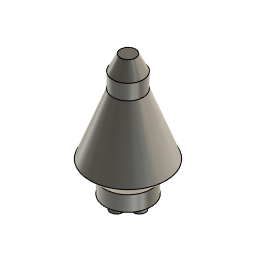
Orbiter v3 (Autodesk Fusion 360 design; units mm, degrees)
Autodesk Fusion 360 part; units mm, degrees
sketch "Sketch1" plane through (0, 0, 0) normal (0, 0, 1) x (1, 0, 0)
  circle A0 centre (0, 0) radius 1500
  constraint coincident A0.centre origin
extrude "Extrude2" add sketch "Sketch1" along normal mid plane 1000 makes body 1
sketch "Sketch4" plane through (0, 0, 0) normal (0, 1, 0) x (1, 0, 0)
  line L0 (0, -500) -> (-1500, -500)
  line L1 (-1500, -500) -> (-2500, -1500)
  line L2 (-2500, -1500) -> (0, -1500)
  line L3 (0, -1500) -> (0, -500)
  line L4 (0, 0) -> (0, -3000)
  constraint horizontal L0
  constraint parallel L0 L2
  constraint perpendicular L0 L3
  constraint coincident L4.start origin
  constraint perpendicular L0 L4
revolve "Revolve1" add sketch "Sketch4" angle 360 about axis through (0, 0, 0) along (0, 0, 1) bodies 1
sketch "Sketch5" plane through (0, 0, 0) normal (0, 1, 0) x (1, 0, 0)
  line L0 (0, -1500) -> (-2500, -1500)
  line L1 (-2500, -1500) -> (-1000, -5500)
  line L2 (-1000, -5500) -> (0, -5500)
  line L3 (0, -5500) -> (0, -1500)
  line L4 (0, 0) -> (0, -6500)
  constraint horizontal L0
  constraint parallel L0 L2
  constraint perpendicular L0 L3
  constraint coincident L4.start origin
  constraint perpendicular L2 L4
revolve "Revolve2" add sketch "Sketch5" angle 360 about axis through (0, 0, 0) along (0, 0, 1) bodies 1
sketch "Sketch6" plane through (0, 0, 5500) normal (0, 0, 1) x (-1, 0, 0)
  circle A0 centre (0, 0) radius 1000
  circle A1 centre (0, 0) radius 1000
  constraint coincident A0.centre A1.centre
extrude "Extrude3" add sketch "Sketch6" along normal blind 1000 bodies 1
sketch "Sketch7" plane through (0, 0, 0) normal (0, 1, 0) x (1, 0, 0)
  line L0 (0, -6500) -> (-1000, -6500)
  line L1 (-1000, -6500) -> (-500, -7500)
  line L2 (-500, -7500) -> (0, -7500)
  line L3 (0, -7500) -> (0, -6500)
  line L4 (0, -6500) -> (0, -8000)
  constraint horizontal L0
  constraint parallel L0 L2
  constraint perpendicular L0 L3
  constraint perpendicular L0 L4
revolve "Revolve3" add sketch "Sketch7" angle 360 about axis through (0, 0, 6500) along (0, 0, 1) bodies 1
sketch "Sketch8" plane through (0, 0, 0) normal (0, 1, 0) x (1, 0, 0)
sketch "Sketch9" plane through (0, 0, 0) normal (0, 1, 0) x (1, 0, 0)
  line L0 (-1000, 500) -> (-500, 500)
  line L1 (-500, 500) -> (-350, 1000)
  line L2 (-350, 1000) -> (-1150, 1000)
  line L3 (-1150, 1000) -> (-1000, 500)
  line L4 (-750, 0) -> (-750, 2500)
  constraint horizontal L0
  constraint parallel L0 L2
  constraint perpendicular L2 L4
revolve "Revolve4" add sketch "Sketch9" angle 360 about axis through (-750, 0, 0) along (0, 0, -1) separate body contours L0 L2 L3 L4 makes body 2
sketch "Sketch10" plane through (0, 0, 0) normal (0, 1, 0) x (1, 0, 0)
  line L0 (0, 0) -> (0, 1000)
  constraint coincident L0.start origin
  constraint vertical L0
sketch "Sketch12" plane through (0, 0, 0) normal (0, 0, 1) x (1, 0, 0)
  line L0 (0, 0) -> (1500, 0)
  constraint coincident L0.start origin
  constraint horizontal L0
pattern_linear "R-Pattern2" count 2 spacing 1500 along (1, 0, 0) of bodies 2 makes body 3
sketch "Sketch13" plane through (0, 0, 0) normal (1, 0, 0) x (0, 1, 0)
  line L0 (-1000, -500) -> (-500, -500)
  line L1 (-500, -500) -> (-350, -1000)
  line L2 (-350, -1000) -> (-1150, -1000)
  line L3 (-1150, -1000) -> (-1000, -500)
  line L4 (-750, -2178.7616) -> (-750, 0)
  constraint horizontal L0
  constraint parallel L0 L2
  constraint perpendicular L0 L4
revolve "Revolve5" add sketch "Sketch13" angle 360 about axis through (0, -750, -2178.7616) along (0, 0, 1) separate body contours L0 L2 L3 L4 makes body 4
sketch "Sketch14" plane through (0, 0, 0) normal (0, 0, 1) x (1, 0, 0)
  line L0 (0, 0) -> (0, 1500)
  constraint coincident L0.start origin
  constraint vertical L0
pattern_linear "R-Pattern3" count 2 spacing 1500 along (0, 1, 0) of bodies 4 makes body 5
sketch "Sketch11" plane through (0, 0, 0) normal (0, 0, 1) x (1, 0, 0)
  line L0 (-750, 0) -> (0, -750)
  line L1 (0, -750) -> (750, 0)
  line L2 (750, 0) -> (0, 750)
  line L3 (0, 750) -> (-750, 0)
  line L4 (0, 1500) -> (0, -1500) construction
  constraint perpendicular L0 L1
  constraint perpendicular L1 L2
  constraint perpendicular L0 L3
  constraint vertical L4
  constraint coincident origin L4
  constraint coincident L0.end L4
pattern_linear "R-Pattern1" [rolled back]
